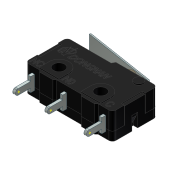
# Autodesk Inventor part: Microswitch Dongnan KW4A (S)
Saved by Autodesk Inventor 2015 (Build 190159000, 159)
## iProperties
Created: 2012-06-23
Part Number: Microswitch Dongnan KW4A (S)
Material: ABS Plastic
Document SubType Name: Modeling
Density: 1.06 g/cm^3
Mass: 1.24115 g
Surface Area: 16.0905 cm^2
Volume: 1.17089 cm^3
Appearance: Smooth - White
Categories: <MemberInstance><Categories><Category DisplayName="" Mnemonic="CABLEANDHARNESS" InternalName="e4a7e005-5e42-4d16-b293-125e7f0d0512"><Category DisplayName="" Mnemonic="CONNECTORS" InternalName="6f634eba-a678-4820-a31d-2c2d5ee6728e"><CategoryParameter DisplayName="" Mnemonic="REFDES" InternalName="c3740e8c-60ab-4d5d-8584-52b73222f2f0"/><Category DisplayName="" Mnemonic="DISCRETEWIRE" InternalName="9a3407de-09b2-4cdb-8c40-9708d5144a28"/></Category></Category></Categories><FamilyTemplate><FamilyTemplateParameters></FamilyTemplateParameters></FamilyTemplate><CategoryParameterMap><ParamToTemplateMap><ParamToTemplate CategoryParameter="//CategoryParameter[@InternalName='c3740e8c-60ab-4d5d-8584-52b73222f2f0']" ConstantValue=""/></ParamToTemplateMap></CategoryParameterMap></MemberInstance>
GlobalPropertyList: <PropertyList/>
Autodesk Inventor part; units mm, degrees
ref_plane "YZ Plane" through (0, 0, 0) normal (1, 0, 0) x (0, 1, 0)
ref_plane "XZ Plane" through (0, 0, 0) normal (0, 1, 0) x (-1, 0, 0)
ref_plane "XY Plane" through (0, 0, 0) normal (0, 0, 1) x (1, 0, 0)
sketch "Sketch1" plane through (0, 0, 0) normal (0, 0, 1) x (1, 0, 0)
  line L0 (-9.9, 5.1) -> (9.9, 5.1)
  line L1 (9.9, 5.1) -> (9.9, -5.1)
  line L2 (9.9, -5.1) -> (-9.9, -5.1)
  line L3 (-9.9, -5.1) -> (-9.9, 5.1)
  line L4 (-6.65, -5.1) -> (-6.25, -5.5)
  line L5 (-6.25, -5.5) -> (-3.25, -5.5)
  line L6 (-3.25, -5.5) -> (-2.85, -5.1)
  line L7 (2.85, -5.1) -> (3.25, -5.5)
  line L8 (3.25, -5.5) -> (6.25, -5.5)
  line L9 (6.25, -5.5) -> (6.65, -5.1)
  line L10 (-9.9, 4.4) -> (0.1, 4.4)
  line L11 (0.1, 4.4) -> (0.5041, 5.1)
  line L12 (4.75, -2.6) -> (-4.75, -2.6) construction
  circle A0 centre (-4.75, -2.6) radius 1.25
  circle A1 centre (4.75, -2.6) radius 1.25
  point P0 (0, 0)
  point P1 (0, 5.1)
  point P2 (9.9, 0)
  point P3 (0, -2.6)
  point P4 (-4.75, -5.5)
  point P5 (4.75, -5.5)
  dimension "d0" = 10.2
  dimension "d1" = 19.8
  dimension "d21" = 0.4
  dimension "d22" = 3
  dimension "d23" = 45
  dimension "d24" = 0.7
  dimension "d25" = 60
  dimension "d26" = 10
  dimension "d27" = 7.7
  dimension "d28" = 9.5
  dimension "d29" = 2.5
  constraints: 26 end point, 6 parallel, 6 point on line, 5 midpoint, 4 vertical alignment, 3 equal length, 2 centre point, 2 coincident, 2 horizontal alignment, 2 perpendicular, 1 collinear, 1 equal radius, 1 horizontal
  measures "d0" distance of L0.end L1.end
  measures "d1" distance of L0.start L0.end
  measures "d21" distance between parallel lines of L2 L8
  measures "d22" distance of L7.end L8.end
  measures "d23" angle of L8 L9
  measures "d24" distance between parallel lines of L0 L10
  measures "d25" angle of L10 L11
  measures "d26" distance of L10.start L10.end
  measures "d27" distance from line of L12.start L0
  measures "d28" distance of L12.start L12.end
  measures "d29" diameter of A0
extrude "Extrusion1" add sketch "Sketch1" along normal mid plane 6 contours L0 L1 L2 L3 L10 L11 | L2 L6 L5 L4 | L9 L8 L7 L2
sketch "Sketch3" plane through (0, 0, 3) normal (0, 0, 1) x (1, 0, 0)
  line L0 (-7, -4.85) -> (-7, -2.6)
  arc A0 (-2.5, -2.6) -> (-7, -2.6) centre (-4.75, -2.6) ccw
  line L1 (-2.5, -2.6) -> (-2.5, -4.85)
  line L2 (-7, -4.85) -> (-2.5, -4.85)
  circle A1 centre (-4.75, -2.6) radius 1.25 projected
  point P0 (0, 0)
  dimension "d13" = 4.5
  constraints: 6 end point, 3 tangent, 2 point on circle, 1 centre point, 1 coincident, 1 parallel, 1 perpendicular, 1 vertical
  measures "d13" distance of L0.start L1.end
extrude "Extrusion2" add sketch "Sketch3" along normal blind 0.25
sketch "Sketch17" plane through (0, 0, 3) normal (0, 0, 1) x (1, 0, 0)
  circle A0 centre (6.9, 3.9) radius 1
  line L0 (9.9, 5.1) -> (9.9, -5.1) projected
  line L1 (9.9, 5.1) -> (0.5041, 5.1) projected
  point P0 (0, 0)
  dimension "d126" = 2
  dimension "d128" = 3
  dimension "d129" = 1.2
  constraints: 1 centre point
  measures "d126" diameter of A0
  measures "d128" distance from line of L0 A0.centre
  measures "d129" distance from line of L1 A0.centre
extrude "Extrusion16" add sketch "Sketch17" along normal up to surface (0.25 mm away)
mirror "Mirror1" about plane through (0, 0, 0) normal (1, 0, 0) of "Extrusion2"
mirror "Mirror2" about plane through (0, 0, 0) normal (0, 0, 1) of "Extrusion2", "Mirror1", "Extrusion16"
sketch "Sketch5" plane through (-2.85, -5.1, 3) normal (0, -1, 0) x (1, 0, 0)
  line L0 (-5.55, -1.4) -> (-4.95, -1.4)
  line L1 (-4.95, -1.4) -> (-4.95, -4.6)
  line L2 (-4.95, -4.6) -> (-5.55, -4.6)
  line L3 (-5.55, -4.6) -> (-5.55, -1.4)
  line L4 (1.75, -1.4) -> (2.35, -1.4)
  line L5 (2.35, -1.4) -> (2.35, -4.6)
  line L6 (2.35, -4.6) -> (1.75, -4.6)
  line L7 (1.75, -4.6) -> (1.75, -1.4)
  line L8 (10.65, -1.4) -> (11.25, -1.4)
  line L9 (11.25, -1.4) -> (11.25, -4.6)
  line L10 (11.25, -4.6) -> (10.65, -4.6)
  line L11 (10.65, -4.6) -> (10.65, -1.4)
  line L12 (-7.05, -6) -> (-7.05, 0) projected
  line L13 (12.75, 0) -> (12.75, -6) projected
  point P0 (2.85, -3)
  point P1 (2.35, -3)
  point P2 (10.65, -3)
  point P3 (-4.95, -3)
  dimension "d30" = 0.6
  dimension "d31" = 3.2
  dimension "d32" = 1.5
  dimension "d33" = 8.8
  dimension "d34" = 1.5
  constraints: 24 end point, 6 parallel, 4 equal length, 3 horizontal, 3 horizontal alignment, 3 midpoint, 3 perpendicular
  measures "d30" distance of L0.start L0.end
  measures "d31" distance of L2.end L0.start
  measures "d32" distance between parallel lines of L12 L3
  measures "d33" distance between parallel lines of L12 L7
  measures "d34" distance between parallel lines of L13 L9
extrude "Extrusion4" add sketch "Sketch5" along normal blind 4.4 separate body
sketch "Sketch6" plane through (8.4, -5.1, 1.6) normal (1, 0, 0) x (0, 0, -1)
  line L0 (0, -4.4) -> (3.2, -4.4) projected
  line L1 (3.2, 0) -> (3.2, -4.4) projected
  line L2 (2.25, -4.4) -> (2.25, -0.9)
  line L3 (2.25, -0.9) -> (3.2, -0.9)
  point P0 (1.6, 5.1)
  dimension "d37" = 3.5
  dimension "d38" = 0.95
  constraints: 4 end point, 2 point on line, 1 parallel, 1 perpendicular
  measures "d37" distance between parallel lines of L0 L3
  measures "d38" distance between parallel lines of L1 L2
extrude "Extrusion5" cut sketch "Sketch6" against normal through all bodies 1 2
mirror "Mirror3" about plane through (0, 0, 0) normal (0, 0, 1) of "Extrusion5" bodies 2
full round fillet "Fillet1" bodies 2 first side at (8, -7.1667, -0.65) centre faces at (8, -9.5, 0.2167) second side at (8, -7.1667, 0.65)
full round fillet "Fillet2" bodies 2 first side at (-0.7, -8.3333, 0.65) centre faces at (-0.9, -9.5, 0.2167) second side at (-0.7, -8.3333, -0.65)
full round fillet "Fillet3" bodies 2 first side at (-8, -8.3333, -0.65) centre faces at (-8.2, -9.5, 0.2167) second side at (-8, -8.3333, 0.65)
fillet "Fillet4" radius 0.1 6 edges at (-8.1, -6, 0.65) (-0.8, -6, 0.65) (8.1, -6, 0.65) (8.1, -6, -0.65) (-0.8, -6, -0.65) (-8.1, -6, -0.65)
sketch "Sketch7" plane through (0, 0, 0) normal (0, 0, 1) x (1, 0, 0)
  line L0 (0.5041, 5.1) -> (9.9, 5.1) projected
  line L1 (1.9, 5.1) -> (1.9, 6.1)
  line L2 (3.9, 5.1) -> (3.9, 6.1)
  arc A0 (3.9, 6.1) -> (1.9, 6.1) centre (2.9, 5.5667) ccw
  line L3 (9.9, 5.1) -> (9.9, -5.1) projected
  point P0 (0, 0)
  dimension "d42" = 2
  dimension "d43" = 6
  dimension "d44" = 1.6
  dimension "d45" = 1
  constraints: 4 end point, 2 point on circle, 2 point on line, 1 centre point, 1 horizontal alignment, 1 parallel, 1 perpendicular
  measures "d42" distance between parallel lines of L1 L2
  measures "d43" distance between parallel lines of L3 L2
  measures "d45" distance of L2.start L2.end
extrude "Extrusion6" add sketch "Sketch7" along normal mid plane 3.6 separate body
sketch "Sketch8" plane through (0.5041, 5.1, 3) normal (0, 1, 0) x (1, 0, 0)
  line L0 (5.5959, 5.1) -> (6.5959, 5.1)
  line L1 (6.5959, 5.1) -> (6.5959, 0.9)
  line L2 (6.5959, 0.9) -> (5.5959, 0.9)
  line L3 (5.5959, 0.9) -> (5.5959, 5.1)
  line L4 (9.3959, 6) -> (9.3959, 0) projected
  point P0 (-0.5041, 3)
  point P1 (6.5959, 3)
  point P2 (9.3959, 3)
  dimension "d48" = 1
  dimension "d49" = 4.2
  dimension "d50" = 2.8
  constraints: 8 end point, 2 midpoint, 2 parallel, 1 horizontal, 1 horizontal alignment, 1 perpendicular
  measures "d48" distance of L0.start L0.end
  measures "d49" distance of L0.end L1.end
  measures "d50" distance between parallel lines of L4 L1
extrude "Extrusion7" cut sketch "Sketch8" against normal blind 1 bodies 1
sketch "Sketch9" plane through (0, 0, 0) normal (0, 0, 1) x (1, 0, 0)
  line L0 (6.9419, 4.1) -> (7.1997, 5.7305)
  line L1 (6.7008, 6.4169) -> (-9.0041, 8.9)
  line L2 (7.1, 4.1) -> (6.1, 4.1) projected
  arc A0 (7.1997, 5.7305) -> (6.7008, 6.4169) centre (6.6071, 5.8242) ccw
  line L3 (0.1, 4.4) -> (-9.9, 4.4) projected
  arc A1 (3.9, 6.1) -> (1.9, 6.1) centre (2.9, 5.5667) ccw projected
  point P0 (0, 0)
  point P1 (7.1, 5.1)
  dimension "d53" = 0.6
  dimension "d54" = 16.5
  dimension "d55" = 4.5
  dimension "d56" = 0.3
  constraints: 4 end point, 2 point on circle, 2 point on line, 2 tangent, 1 centre point, 1 perpendicular
  measures "d53" radius of A0
  measures "d54" distance from line of L1.end L0
  measures "d55" distance from line of L1.end L3
  measures "d56" distance edge to line of A1 L1
surface extrude "ExtrusionSrf1" sketch "Sketch9" along normal mid plane 4.1 shown no curves L0 A0 L1
thicken "Thicken1" operation new thickness 0.3 both sides no extend neighbours no toward (-0.9877298, 0.1561724, 0) faces at (7.0278, 4.6435, -0.6833) (7.1495, 6.0806, 0.6833) (1.4658, 7.2446, -0.6833)
fillet "Fillet5" radius 0.8 4 edges at (-9.9, 4.4, 0) (-9.9, -5.1, 0) (9.9, -5.1, 0) (9.9, 5.1, 0)
ref_plane "Work Plane1" through (0, 0, -1) normal (0, 0, 1) x (1, 0, 0)
split body "Split1" result two bodies by plane through (0, 0, -1) normal (0, 0, 1) bodies 1 first body at (-4.5331, 2.4803, -0.5)
sketch "Sketch10" plane through (0.1, 4.4, -1) normal (0, 0, -1) x (-1, 0, 0)
  line L0 (10, -8.7) -> (10, -0.8) projected
  line L1 (9.3, -2) -> (10, -2)
  line L2 (10, -2) -> (10, -6.8)
  line L3 (10, -6.8) -> (9.3, -6.8)
  line L4 (9.3, -6.8) -> (9.3, -2)
  line L5 (9.2, 0) -> (0, 0) projected
  point P0 (0.1, -4.4)
  dimension "d62" = 0.7
  dimension "d63" = 2
  dimension "d64" = 4.8
  constraints: 8 end point, 2 parallel, 1 horizontal, 1 perpendicular, 1 point on line
  measures "d62" distance between parallel lines of L2 L4
  measures "d63" distance between parallel lines of L5 L1
  measures "d64" distance of L3.end L1.start
extrude "Extrusion8" cut sketch "Sketch10" against normal through all bodies 5
sketch "Sketch11" plane through (0, 0, 0) normal (0, 1, 0) x (-1, 0, 0)
  line L0 (9.2, 0.1) -> (9.6, 0.1)
  line L1 (9.6, 0.1) -> (9.6, -0.7)
  line L2 (9.6, -0.7) -> (8.9, -2.2)
  line L3 (8.9, -2.2) -> (8.6, -2.2)
  line L4 (9.2, 3) -> (9.9, 3) projected
  line L5 (9.2, -1) -> (9.2, 3) projected
  line L6 (9.9, 3) -> (9.9, -1) projected
  line L7 (8.6, -2.2) -> (8.6, -1)
  line L8 (8.6, -1) -> (9.2, -1)
  point P0 (0, 0)
  dimension "d68" = 5.2
  dimension "d69" = 2.9
  dimension "d70" = 0.8
  dimension "d72" = 0.3
  dimension "d73" = 1
  dimension "d74" = 0.3
  constraints: 12 end point, 2 parallel, 1 perpendicular, 1 point on line, 1 vertical
  measures "d68" distance between parallel lines of L3 L4
  measures "d69" distance between parallel lines of L4 L0
  measures "d70" distance of L0.end L1.end
  measures "d72" distance between parallel lines of L1 L6
  measures "d73" distance from line of L6 L2.end
  measures "d74" distance of L2.end L3.end
extrude "Extrusion9" add sketch "Sketch11" along normal mid plane 1.3 bodies 5
sketch "Sketch12" plane through (-9.1, 4.4, -1) normal (0, 0, 1) x (1, 0, 0)
  line L0 (-0.8, -8.7) -> (-0.8, -0.8) projected
  line L1 (-0.8, -2.05) -> (-0.1, -2.05)
  line L2 (-0.1, -2.05) -> (-0.1, -6.75)
  line L3 (-0.1, -6.75) -> (-0.8, -6.75)
  line L4 (-0.8, -6.75) -> (-0.8, -2.05)
  line L5 (-0.5, -3.75) -> (-0.5, -5.05) projected
  point P0 (9.1, -4.4)
  point P1 (-0.1, -4.4)
  point P2 (-0.8, -4.4)
  point P3 (-0.5, -4.4)
  dimension "d77" = 0.7
  dimension "d78" = 4.7
  constraints: 8 end point, 3 midpoint, 2 horizontal alignment, 2 parallel, 1 horizontal, 1 perpendicular, 1 point on line
  measures "d77" distance of L1.start L1.end
  measures "d78" distance of L1.end L2.end
extrude "Extrusion10" add sketch "Sketch12" along normal blind 3.8 bodies 6
sketch "Sketch13" plane through (0, 0, -3) normal (0, 0, -1) x (-1, 0, 0)
  line L0 (9.9, 3.6) -> (9.9, -4.3) projected
  line L1 (9.9, 0.65) -> (8.9, 0.65)
  line L2 (8.9, 0.65) -> (8.9, -0.65)
  line L3 (8.9, -0.65) -> (9.9, -0.65)
  line L4 (9.9, -0.65) -> (9.9, 0.65)
  line L5 (9.9, -2.35) -> (9.9, 2.35) projected
  point P0 (0, 0)
  point P1 (9.9, 0)
  point P2 (9.9, -0.35)
  point P3 (9.9, 0)
  dimension "d81" = 1.3
  dimension "d82" = 1
  constraints: 8 end point, 3 midpoint, 2 parallel, 1 coincident, 1 horizontal, 1 perpendicular, 1 point on line
  measures "d81" distance of L1.end L2.end
  measures "d82" distance of L2.end L3.end
extrude "Extrusion11" cut sketch "Sketch13" against normal blind 3.1 bodies 6
sketch "Sketch14" plane through (-8.9, -0.65, -3) normal (-1, 0, 0) x (0, 0, 1)
  line L0 (2, 1.3) -> (2, 0) projected
  line L1 (0, 1.3) -> (2, 1.3) projected
  line L2 (0, 0) -> (0, 1.3) projected
  line L3 (0, 0) -> (2, 0) projected
  line L4 (2, 1.3) -> (0.7, 1.3)
  line L5 (0.7, 1.3) -> (0.7, 0)
  line L6 (0.7, 0) -> (2, 0)
  line L7 (2, 0) -> (2, 1.3)
  point P0 (3, 0.65)
  dimension "d85" = 0.7
  constraints: 8 end point, 2 parallel, 1 horizontal, 1 perpendicular, 1 point on line
  measures "d85" distance between parallel lines of L2 L5
extrude "Extrusion12" cut sketch "Sketch14" against normal blind 1 contours L0 L3 L5 L1 bodies 6
mirror "Mirror4" about plane through (0, 0, 0) normal (1, 0, 0) of "Extrusion8", "Extrusion9" bodies 5
mirror "Mirror5" about plane through (0, 0, 0) normal (1, 0, 0) of "Extrusion10", "Extrusion11", "Extrusion12" bodies 6
sketch "Sketch15" plane through (0, 0, 3) normal (0, 0, 1) x (1, 0, 0)
  line L0 (-9.6, -3.1) -> (-7.0718, -3.1) construction
  line L1 (-7.0718, -3.1) -> (-7.0718, -5.3594) construction
  line L2 (-7.0718, -5.3594) -> (-9.6, -5.3594) construction
  line L3 (-9.6, -5.3594) -> (-9.6, -3.1) construction
  line L4 (-2.3, -3.1) -> (0.2282, -3.1) construction
  line L5 (0.2282, -3.1) -> (0.2282, -5.3594) construction
  line L6 (0.2282, -5.3594) -> (-2.3, -5.3594) construction
  line L7 (-2.3, -5.3594) -> (-2.3, -3.1) construction
  line L8 (7.5, -5.3594) -> (7.5, -3.1) construction
  line L9 (7.5, -3.1) -> (10.0282, -3.1) construction
  line L10 (10.0282, -3.1) -> (10.0282, -5.3594) construction
  line L11 (10.0282, -5.3594) -> (7.5, -5.3594) construction
  line L12 (-6.65, -5.1) -> (-9.1, -5.1) projected
  line L13 (-9.9, -4.3) -> (-9.9, -2.4) projected
  line L14 (-6.1061, 1.9) -> (2.8193, 1.9) construction
  line L15 (2.8193, 1.9) -> (2.8193, 0.5) construction
  line L16 (2.8193, 0.5) -> (-6.1061, 0.5) construction
  line L17 (-6.1061, 0.5) -> (-6.1061, 1.9) construction
  line L18 (-8.2, 0.6) -> (-7.85, 0.6)
  line L19 (-7.85, 0.6) -> (-7.5869, 2.0924)
  line L20 (-7.5869, 2.0924) -> (-7.3061, 0.5)
  line L21 (-7.3061, 0.5) -> (-6.8061, 0.5)
  line L22 (-6.8061, 0.5) -> (-6.5436, 3.5)
  line L23 (-6.5436, 3.5) -> (-7.0746, 1.2)
  line L24 (-7.0746, 1.2) -> (-7.5569, 3)
  line L25 (-7.5569, 3) -> (-8.2, 0.6)
  arc A0 (-6.5495, 2.7981) -> (-8.3, 1.85) centre (-6.3326, 0.3075) ccw
  arc A1 (-6.0803, 2.0379) -> (-6.5495, 2.7981) centre (-6.5061, 2.3) ccw
  arc A2 (-8.3, 0.85) -> (-6.0803, 2.0379) centre (-8.2093, 3.3484) ccw
  line L26 (-8.3, 1.85) -> (-8.3, 0.85)
  arc A3 (-6.5581, 2.8977) -> (-8.4, 1.8841) centre (-6.3326, 0.3075) ccw
  arc A4 (-5.9951, 1.9855) -> (-6.5581, 2.8977) centre (-6.5061, 2.3) ccw
  arc A5 (-8.4, 0.7554) -> (-5.9951, 1.9855) centre (-8.2093, 3.3484) ccw
  line L27 (-8.4, 0.7554) -> (-8.4, 1.8841)
  line L28 (-9.2, 2.4) -> (-9.2, -2.4) projected
  line L29 (-9.472, -4.6263) -> (-9.472, -3.1263)
  line L30 (-9.472, -3.1263) -> (-9.3096, -3.1263)
  line L31 (-9.3096, -3.1263) -> (-8.6785, -4.3039)
  line L32 (-8.6785, -4.3039) -> (-8.6785, -3.1263)
  line L33 (-8.6785, -3.1263) -> (-8.5264, -3.1263)
  line L34 (-8.5264, -3.1263) -> (-8.5264, -4.6263)
  line L35 (-8.5264, -4.6263) -> (-8.6888, -4.6263)
  line L36 (-8.6888, -4.6263) -> (-9.3199, -3.4487)
  line L37 (-9.3199, -3.4487) -> (-9.3199, -4.6263)
  line L38 (-9.3199, -4.6263) -> (-9.472, -4.6263)
  line L39 (-7.4049, -4.0992) -> (-7.246, -4.1495)
  spline S0 degree 2 poles (-7.246, -4.1495) (-7.2963, -4.3942) (-7.5558, -4.6514) (-7.7433, -4.6514) knots 0 0 0 1 2 2 2
  spline S1 degree 2 poles (-7.7433, -4.6514) (-7.9365, -4.6514) (-8.18, -4.4537) (-8.3069, -4.0798) (-8.3069, -3.8649) knots 0 0 0 1 2 3 3 3
  spline S2 degree 2 poles (-8.3069, -3.8649) (-8.3069, -3.6305) (-8.164, -3.2806) (-7.8988, -3.1) (-7.741, -3.1) knots 0 0 0 1 2 3 3 3
  spline S3 degree 2 poles (-7.741, -3.1) (-7.5604, -3.1) (-7.3146, -3.3298) (-7.2665, -3.5367) knots 0 0 0 1 2 2 2
  line L40 (-7.2665, -3.5367) -> (-7.4232, -3.5836)
  spline S4 degree 2 poles (-7.4232, -3.5836) (-7.4655, -3.4201) (-7.6232, -3.2704) (-7.7444, -3.2704) knots 0 0 0 1 2 2 2
  spline S5 degree 2 poles (-7.7444, -3.2704) (-7.8828, -3.2704) (-8.068, -3.4361) (-8.1434, -3.7151) (-8.1434, -3.8637) knots 0 0 0 1 2 3 3 3
  spline S6 degree 2 poles (-8.1434, -3.8637) (-8.1434, -4.0546) (-8.0543, -4.3405) (-7.8656, -4.4811) (-7.7559, -4.4811) knots 0 0 0 1 2 3 3 3
  spline S7 degree 2 poles (-7.7559, -4.4811) (-7.6221, -4.4811) (-7.438, -4.289) (-7.4049, -4.0992) knots 0 0 0 1 2 2 2
  line L41 (-2.172, -4.6057) -> (-2.172, -3.1057)
  line L42 (-2.172, -3.1057) -> (-2.0096, -3.1057)
  line L43 (-2.0096, -3.1057) -> (-1.3785, -4.2833)
  line L44 (-1.3785, -4.2833) -> (-1.3785, -3.1057)
  line L45 (-1.3785, -3.1057) -> (-1.2264, -3.1057)
  line L46 (-1.2264, -3.1057) -> (-1.2264, -4.6057)
  line L47 (-1.2264, -4.6057) -> (-1.3888, -4.6057)
  line L48 (-1.3888, -4.6057) -> (-2.0199, -3.4281)
  line L49 (-2.0199, -3.4281) -> (-2.0199, -4.6057)
  line L50 (-2.0199, -4.6057) -> (-2.172, -4.6057)
  spline S8 degree 2 poles (-1.0207, -3.866) (-1.0207, -3.5996) (-0.9326, -3.2749) (-0.76, -3.1) (-0.6296, -3.1) knots 0 0 0 1 2 3 3 3
  spline S9 degree 2 poles (-0.6296, -3.1) (-0.5336, -3.1) (-0.3873, -3.1972) (-0.2924, -3.3801) (-0.2386, -3.6431) (-0.2386, -3.866) knots 0 0 0 1 2 3 4 4 4
  spline S10 degree 2 poles (-0.2386, -3.866) (-0.2386, -4.1301) (-0.3255, -4.4548) (-0.4982, -4.6309) (-0.6296, -4.6309) knots 0 0 0 1 2 3 3 3
  spline S11 degree 2 poles (-0.6296, -4.6309) (-0.8034, -4.6309) (-0.9018, -4.4765) knots 0 0 0 1 1 1
  spline S12 degree 2 poles (-0.9018, -4.4765) (-1.0207, -4.2879) (-1.0207, -3.866) knots 0 0 0 1 1 1
  spline S13 degree 2 poles (-0.8697, -3.866) (-0.8697, -4.2364) (-0.7314, -4.48) (-0.6296, -4.48) knots 0 0 0 1 2 2 2
  spline S14 degree 2 poles (-0.6296, -4.48) (-0.5279, -4.48) (-0.3896, -4.2353) (-0.3896, -3.866) knots 0 0 0 1 2 2 2
  spline S15 degree 2 poles (-0.3896, -3.866) (-0.3896, -3.4956) (-0.5279, -3.2521) (-0.6308, -3.2521) knots 0 0 0 1 2 2 2
  spline S16 degree 2 poles (-0.6308, -3.2521) (-0.7325, -3.2521) (-0.7943, -3.3595) knots 0 0 0 1 1 1
  spline S17 degree 2 poles (-0.7943, -3.3595) (-0.8697, -3.4967) (-0.8697, -3.866) knots 0 0 0 1 1 1
  spline S18 degree 2 poles (-4.6762, 1.1955) (-4.7386, 1.0106) (-4.9891, 0.713) (-5.1434, 0.6299) knots 0 0 0 1 2 2 2
  spline S19 degree 2 poles (-5.1434, 0.6299) (-5.2681, 0.5653) (-5.4945, 0.5216) (-5.6586, 0.5216) knots 0 0 0 1 2 2 2
  line L51 (-5.6586, 0.5216) -> (-5.9693, 0.5216)
  line L52 (-5.9693, 0.5216) -> (-5.5109, 1.8716)
  line L53 (-5.5109, 1.8716) -> (-5.2035, 1.8716)
  spline S20 degree 2 poles (-5.2035, 1.8716) (-5.0132, 1.8716) (-4.8152, 1.8147) (-4.7561, 1.7643) knots 0 0 0 1 2 2 2
  spline S21 degree 2 poles (-4.7561, 1.7643) (-4.6554, 1.6779) (-4.6084, 1.3924) (-4.6762, 1.1955) knots 0 0 0 1 2 2 2
  spline S22 degree 2 poles (-4.8622, 1.1976) (-4.8097, 1.353) (-4.8381, 1.5729) (-4.918, 1.6353) knots 0 0 0 1 2 2 2
  spline S23 degree 2 poles (-4.918, 1.6353) (-4.9749, 1.6779) (-5.1259, 1.7162) (-5.2473, 1.7162) knots 0 0 0 1 2 2 2
  line L54 (-5.2473, 1.7162) -> (-5.384, 1.7162)
  line L55 (-5.384, 1.7162) -> (-5.7374, 0.6769)
  line L56 (-5.7374, 0.6769) -> (-5.6007, 0.6769)
  spline S24 degree 2 poles (-5.6007, 0.6769) (-5.4803, 0.6769) (-5.2878, 0.7152) (-5.1959, 0.7666) knots 0 0 0 1 2 2 2
  spline S25 degree 2 poles (-5.1959, 0.7666) (-5.081, 0.8301) (-4.9158, 1.0401) (-4.8622, 1.1976) knots 0 0 0 1 2 2 2
  spline S26 degree 2 poles (-3.3492, 1.7173) (-3.3022, 1.6276) (-3.3065, 1.365) (-3.3634, 1.1966) knots 0 0 0 1 2 2 2
  spline S27 degree 2 poles (-3.3634, 1.1966) (-3.4192, 1.0325) (-3.5932, 0.7666) (-3.7026, 0.6769) knots 0 0 0 1 2 2 2
  spline S28 degree 2 poles (-3.7026, 0.6769) (-3.8174, 0.5828) (-4.068, 0.4931) (-4.2003, 0.4931) knots 0 0 0 1 2 2 2
  spline S29 degree 2 poles (-4.2003, 0.4931) (-4.3371, 0.4931) (-4.5252, 0.5861) (-4.5723, 0.6769) knots 0 0 0 1 2 2 2
  spline S30 degree 2 poles (-4.5723, 0.6769) (-4.6204, 0.7666) (-4.6139, 1.0303) (-4.557, 1.1966) knots 0 0 0 1 2 2 2
  spline S31 degree 2 poles (-4.557, 1.1966) (-4.499, 1.3661) (-4.3272, 1.6243) (-4.2178, 1.7173) knots 0 0 0 1 2 2 2
  spline S32 degree 2 poles (-4.2178, 1.7173) (-4.1095, 1.807) (-3.8579, 1.9) (-3.7222, 1.9) knots 0 0 0 1 2 2 2
  spline S33 degree 2 poles (-3.7222, 1.9) (-3.5844, 1.9) (-3.3962, 1.8037) (-3.3492, 1.7173) knots 0 0 0 1 2 2 2
  spline S34 degree 2 poles (-3.5505, 1.1966) (-3.5056, 1.33) (-3.4936, 1.5368) (-3.522, 1.6046) knots 0 0 0 1 2 2 2
  spline S35 degree 2 poles (-3.522, 1.6046) (-3.5527, 1.6746) (-3.6796, 1.7447) (-3.7737, 1.7447) knots 0 0 0 1 2 2 2
  spline S36 degree 2 poles (-3.7737, 1.7447) (-3.8721, 1.7447) (-4.0406, 1.6768) (-4.1205, 1.6046) knots 0 0 0 1 2 2 2
  spline S37 degree 2 poles (-4.1205, 1.6046) (-4.1981, 1.5357) (-4.3261, 1.3278) (-4.3699, 1.1966) knots 0 0 0 1 2 2 2
  spline S38 degree 2 poles (-4.3699, 1.1966) (-4.4607, 0.9307) (-4.3338, 0.6485) (-4.1467, 0.6485) knots 0 0 0 1 2 2 2
  spline S39 degree 2 poles (-4.1467, 0.6485) (-3.9586, 0.6485) (-3.6413, 0.9307) (-3.5505, 1.1966) knots 0 0 0 1 2 2 2
  line L57 (-2.4302, 0.5216) -> (-2.6315, 0.5216)
  line L58 (-2.6315, 0.5216) -> (-2.8328, 1.6856)
  line L59 (-2.8328, 1.6856) -> (-3.2289, 0.5216)
  line L60 (-3.2289, 0.5216) -> (-3.3962, 0.5216)
  line L61 (-3.3962, 0.5216) -> (-2.9378, 1.8716)
  line L62 (-2.9378, 1.8716) -> (-2.6829, 1.8716)
  line L63 (-2.6829, 1.8716) -> (-2.5024, 0.8027)
  line L64 (-2.5024, 0.8027) -> (-2.1392, 1.8716)
  line L65 (-2.1392, 1.8716) -> (-1.9718, 1.8716)
  line L66 (-1.9718, 1.8716) -> (-2.4302, 0.5216)
  spline S40 degree 2 poles (-1.5999, 0.4953) (-1.7432, 0.4953) (-1.9511, 0.5828) (-2.0069, 0.6714) knots 0 0 0 1 2 2 2
  spline S41 degree 2 poles (-2.0069, 0.6714) (-2.0616, 0.7611) (-2.0616, 1.0259) (-2.0036, 1.1976) knots 0 0 0 1 2 2 2
  spline S42 degree 2 poles (-2.0036, 1.1976) (-1.9478, 1.3607) (-1.7684, 1.6188) (-1.6524, 1.7107) knots 0 0 0 1 2 2 2
  spline S43 degree 2 poles (-1.6524, 1.7107) (-1.5397, 1.7994) (-1.2662, 1.8956) (-1.1229, 1.8956) knots 0 0 0 1 2 2 2
  spline S44 degree 2 poles (-1.1229, 1.8956) (-1.0551, 1.8956) (-0.9358, 1.8759) (-0.8855, 1.8584) knots 0 0 0 1 2 2 2
  spline S45 degree 2 poles (-0.8855, 1.8584) (-0.8439, 1.8453) (-0.7487, 1.7972) (-0.7203, 1.7797) knots 0 0 0 1 2 2 2
  line L67 (-0.7203, 1.7797) -> (-0.7936, 1.563)
  line L68 (-0.7936, 1.563) -> (-0.81, 1.563)
  spline S46 degree 2 poles (-0.81, 1.563) (-0.833, 1.5926) (-0.8866, 1.6462) (-0.9413, 1.6768) knots 0 0 0 1 2 2 2
  spline S47 degree 2 poles (-0.9413, 1.6768) (-0.9861, 1.7042) (-1.1152, 1.7403) (-1.1973, 1.7403) knots 0 0 0 1 2 2 2
  spline S48 degree 2 poles (-1.1973, 1.7403) (-1.392, 1.7403) (-1.7323, 1.4471) (-1.8143, 1.2031) knots 0 0 0 1 2 2 2
  spline S49 degree 2 poles (-1.8143, 1.2031) (-1.8603, 1.0675) (-1.8657, 0.864) (-1.8307, 0.794) knots 0 0 0 1 2 2 2
  spline S50 degree 2 poles (-1.8307, 0.794) (-1.7957, 0.7239) (-1.6568, 0.6506) (-1.5539, 0.6506) knots 0 0 0 1 2 2 2
  spline S51 degree 2 poles (-1.5539, 0.6506) (-1.4784, 0.6506) (-1.3198, 0.6725) (-1.2607, 0.6944) knots 0 0 0 1 2 2 2
  line L69 (-1.2607, 0.6944) -> (-1.1426, 1.0434)
  line L70 (-1.1426, 1.0434) -> (-1.4555, 1.0434)
  line L71 (-1.4555, 1.0434) -> (-1.4019, 1.2009)
  line L72 (-1.4019, 1.2009) -> (-0.9118, 1.2009)
  line L73 (-0.9118, 1.2009) -> (-1.112, 0.6113)
  spline S52 degree 2 poles (-1.112, 0.6113) (-1.1513, 0.5959) (-1.2826, 0.5489) (-1.3373, 0.5347) knots 0 0 0 1 2 2 2
  spline S53 degree 2 poles (-1.3373, 0.5347) (-1.4106, 0.515) (-1.5244, 0.4953) (-1.5999, 0.4953) knots 0 0 0 1 2 2 2
  line L74 (0.0488, 0.5216) -> (-0.1525, 0.5216)
  line L75 (-0.1525, 0.5216) -> (-0.3538, 1.6856)
  line L76 (-0.3538, 1.6856) -> (-0.7498, 0.5216)
  line L77 (-0.7498, 0.5216) -> (-0.9172, 0.5216)
  line L78 (-0.9172, 0.5216) -> (-0.4588, 1.8716)
  line L79 (-0.4588, 1.8716) -> (-0.2039, 1.8716)
  line L80 (-0.2039, 1.8716) -> (-0.0234, 0.8027)
  line L81 (-0.0234, 0.8027) -> (0.3398, 1.8716)
  line L82 (0.3398, 1.8716) -> (0.5072, 1.8716)
  line L83 (0.5072, 1.8716) -> (0.0488, 0.5216)
  line L84 (0.1768, 0.5216) -> (1.0903, 1.8716)
  line L85 (1.0903, 1.8716) -> (1.3113, 1.8716)
  line L86 (1.3113, 1.8716) -> (1.308, 0.5216)
  line L87 (1.308, 0.5216) -> (1.1187, 0.5216)
  line L88 (1.1187, 0.5216) -> (1.1242, 0.899)
  line L89 (1.1242, 0.899) -> (0.6089, 0.899)
  line L90 (0.6089, 0.899) -> (0.3584, 0.5216)
  line L91 (0.3584, 0.5216) -> (0.1768, 0.5216)
  line L92 (1.1264, 1.0521) -> (1.134, 1.6878)
  line L93 (1.134, 1.6878) -> (0.7107, 1.0521)
  line L94 (0.7107, 1.0521) -> (1.1264, 1.0521)
  line L95 (2.402, 0.5216) -> (2.2007, 0.5216)
  line L96 (2.2007, 0.5216) -> (1.9994, 1.6856)
  line L97 (1.9994, 1.6856) -> (1.6034, 0.5216)
  line L98 (1.6034, 0.5216) -> (1.436, 0.5216)
  line L99 (1.436, 0.5216) -> (1.8944, 1.8716)
  line L100 (1.8944, 1.8716) -> (2.1493, 1.8716)
  line L101 (2.1493, 1.8716) -> (2.3298, 0.8027)
  line L102 (2.3298, 0.8027) -> (2.693, 1.8716)
  line L103 (2.693, 1.8716) -> (2.8604, 1.8716)
  line L104 (2.8604, 1.8716) -> (2.402, 0.5216)
  line L105 (8.4855, -4.0992) -> (8.6444, -4.1495)
  spline S54 degree 2 poles (8.6444, -4.1495) (8.5941, -4.3942) (8.3346, -4.6514) (8.1471, -4.6514) knots 0 0 0 1 2 2 2
  spline S55 degree 2 poles (8.1471, -4.6514) (7.9539, -4.6514) (7.7104, -4.4537) (7.5835, -4.0798) (7.5835, -3.8649) knots 0 0 0 1 2 3 3 3
  spline S56 degree 2 poles (7.5835, -3.8649) (7.5835, -3.6305) (7.7264, -3.2806) (7.9916, -3.1) (8.1494, -3.1) knots 0 0 0 1 2 3 3 3
  spline S57 degree 2 poles (8.1494, -3.1) (8.33, -3.1) (8.5758, -3.3298) (8.6239, -3.5367) knots 0 0 0 1 2 2 2
  line L106 (8.6239, -3.5367) -> (8.4672, -3.5836)
  spline S58 degree 2 poles (8.4672, -3.5836) (8.4249, -3.4201) (8.2671, -3.2704) (8.146, -3.2704) knots 0 0 0 1 2 2 2
  spline S59 degree 2 poles (8.146, -3.2704) (8.0076, -3.2704) (7.8224, -3.4361) (7.747, -3.7151) (7.747, -3.8637) knots 0 0 0 1 2 3 3 3
  spline S60 degree 2 poles (7.747, -3.8637) (7.747, -4.0546) (7.8361, -4.3405) (8.0248, -4.4811) (8.1345, -4.4811) knots 0 0 0 1 2 3 3 3
  spline S61 degree 2 poles (8.1345, -4.4811) (8.2683, -4.4811) (8.4524, -4.289) (8.4855, -4.0992) knots 0 0 0 1 2 2 2
  point P0 (0, 0)
  dimension "d88" = 2
  dimension "d89" = 0.3
  dimension "d90" = 7.6
  dimension "d91" = 17.4
  dimension "d92" = 0.5
  dimension "d93" = 0.35
  dimension "d94" = 0.1
  dimension "d95" = 95
  dimension "d96" = 3
  dimension "d97" = 8
  dimension "d99" = 100
  dimension "d100" = 100
  dimension "d101" = 75
  dimension "d102" = 0.7
  dimension "d103" = 0.5
  dimension "d104" = 28
  dimension "d105" = 1.4
  dimension "d106" = 0.7
  dimension "d107" = 1.8
  dimension "d108" = 0.5
  dimension "d109" = 2.5
  dimension "d110" = 2.5
  dimension "d111" = 0.1
  dimension "d112" = 1
  dimension "d113" = 0.35
  dimension "d114" = 0.3
  dimension "d115" = 0.1
  dimension "d116" = 0.8
  dimension "d117" = 5.6
  constraints: 20 end point, 12 point on circle, 6 centre point, 3 horizontal alignment, 2 perpendicular, 2 tangent, 1 horizontal, 1 parallel, 11 other
  measures "d88" distance between parallel lines of L12 L0
  measures "d89" distance between parallel lines of L3 L13
  measures "d90" distance between parallel lines of L13 L7
  measures "d91" distance between parallel lines of L13 L8
  measures "d92" distance of L20.end L21.end
  measures "d93" distance of L18.start L18.end
  measures "d94" distance between parallel lines of L18 L21
  measures "d95" angle of L22 L21
  measures "d96" distance from line of L22.end L21
  measures "d97" angle of L22 L23
  measures "d99" angle of L21 L20
  measures "d100" angle of L18 L19
  measures "d101" angle of L18 L25
  measures "d102" distance from line of L21 L23.end
  measures "d103" vertical distance of L24.end L22.end
  measures "d104" angle of L23 L24
  measures "d105" distance of L16.end L14.start
  measures "d106" distance from line of L21.end L17
  measures "d107" distance from line of L21 A1.centre
  measures "d108" radius of A1
  measures "d109" radius of A0
  measures "d110" radius of A2
  measures "d111" distance from line of L18.start L26
  measures "d112" distance of L26.start L26.end
  measures "d113" distance from line of L21 L26.end
  measures "d114" horizontal distance of L21.end A1.centre
  measures "d115" radial gap between concentric circles of A1 A4
  measures "d116" distance between parallel lines of L28 L27
  measures "d117" distance between parallel lines of L12 L16
extrude "Extrusion13" add sketch "Sketch15" along normal blind 0.1 contours L25 A5 L19 L18 | A5 L27 A3 L25 A0 L26 A2 | L25 A2 L19 A5 | L19 A2 L20 A5 | L25 A0 L24 L23 L22 A2 L20 L19 | A5 L22 L21 L20 | L20 A2 L22 A5 | L25 A3 L24 A0 | L22 A2 A1 A0 A3 A4 A5 | L25 L24 A3 | L24 A3 L23 A0 | L23 A3 L22 A0 | L23 L22 A3 | L29 L30 L31 L32 L33 L34 L35 L36 L37 L38 | L39 S0 S1 S2 S3 L40 S4 S5 S6 S7 | L41 L42 L43 L44 L45 L46 L47 L48 L49 L50 | S8 S9 S10 S11 S12 | S18 S19 L51 L52 L53 S20 S21 | S26 S27 S28 S29 S30 S31 S32 S33 | L57 L58 L59 L60 L61 L62 L63 L64 L65 L66 | S40 S41 S42 S43 S44 S45 L67 L68 S46 S47 S48 S49 S50 S51 L69 L70 L71 L72 L73 S52 S53 | L74 L75 L76 L77 L78 L79 L80 L81 L82 L83 | L84 L85 L86 L87 L88 L89 L90 L91 | L95 L96 L97 L98 L99 L100 L101 L102 L103 L104 | L105 S54 S55 S56 S57 L106 S58 S59 S60 S61 bodies 5
extrude "Extrusion14" add sketch "Sketch15" along normal up to surface (0.1 mm away) contours L25 A5 L19 L18 | L25 A2 L19 A5 | L25 A0 L24 L23 L22 A2 L20 L19 | A5 L22 L21 L20 | L20 A2 L22 A5 | L25 A3 L24 A0 | L25 L24 A3 | L23 A3 L22 A0 | L23 L22 A3 bodies 5
sketch "Sketch16" plane through (0, 0, -3) normal (0, 0, -1) x (-1, 0, 0)
  line L0 (-5.4, 4.6) -> (15.1547, 4.6) construction
  line L1 (15.1547, 4.6) -> (15.1547, -0.0232) construction
  line L2 (15.1547, -0.0232) -> (-5.4, -0.0232) construction
  line L3 (-5.4, -0.0232) -> (-5.4, 4.6) construction
  line L4 (-9.1, 5.1) -> (-0.5041, 5.1) projected
  line L5 (-9.9, 0.65) -> (-9.9, 4.3) projected
  line L6 (-4.7363, 3.5554) -> (-4.8741, 3.5554)
  line L7 (-4.8741, 3.5554) -> (-5.1658, 4.0206)
  line L8 (-5.1658, 4.0206) -> (-5.2128, 3.9549)
  line L9 (-5.2128, 3.9549) -> (-5.2128, 3.5554)
  line L10 (-5.2128, 3.5554) -> (-5.319, 3.5554)
  line L11 (-5.319, 3.5554) -> (-5.319, 4.5554)
  line L12 (-5.319, 4.5554) -> (-5.2128, 4.5554)
  line L13 (-5.2128, 4.5554) -> (-5.2128, 4.0951)
  line L14 (-5.2128, 4.0951) -> (-4.8854, 4.5554)
  line L15 (-4.8854, 4.5554) -> (-4.7558, 4.5554)
  line L16 (-4.7558, 4.5554) -> (-5.0864, 4.1089)
  line L17 (-5.0864, 4.1089) -> (-4.7363, 3.5554)
  line L18 (-3.7752, 4.5554) -> (-3.9762, 3.5554)
  line L19 (-3.9762, 3.5554) -> (-4.0961, 3.5554)
  line L20 (-4.0961, 3.5554) -> (-4.259, 4.3853)
  line L21 (-4.259, 4.3853) -> (-4.4178, 3.5554)
  line L22 (-4.4178, 3.5554) -> (-4.5345, 3.5554)
  line L23 (-4.5345, 3.5554) -> (-4.7395, 4.5554)
  line L24 (-4.7395, 4.5554) -> (-4.6301, 4.5554)
  line L25 (-4.6301, 4.5554) -> (-4.4689, 3.724)
  line L26 (-4.4689, 3.724) -> (-4.3092, 4.5554)
  line L27 (-4.3092, 4.5554) -> (-4.2015, 4.5554)
  line L28 (-4.2015, 4.5554) -> (-4.0394, 3.7159)
  line L29 (-4.0394, 3.7159) -> (-3.8797, 4.5554)
  line L30 (-3.8797, 4.5554) -> (-3.7752, 4.5554)
  line L31 (-3.1885, 3.899) -> (-3.2833, 3.899)
  line L32 (-3.2833, 3.899) -> (-3.2833, 3.5554)
  line L33 (-3.2833, 3.5554) -> (-3.3862, 3.5554)
  line L34 (-3.3862, 3.5554) -> (-3.3862, 3.899)
  line L35 (-3.3862, 3.899) -> (-3.7395, 3.899)
  line L36 (-3.7395, 3.899) -> (-3.7395, 4.04)
  line L37 (-3.7395, 4.04) -> (-3.3822, 4.5554)
  line L38 (-3.3822, 4.5554) -> (-3.2833, 4.5554)
  line L39 (-3.2833, 4.5554) -> (-3.2833, 4.0068)
  line L40 (-3.2833, 4.0068) -> (-3.1885, 4.0068)
  line L41 (-3.1885, 4.0068) -> (-3.1885, 3.899)
  line L42 (-3.3862, 4.0068) -> (-3.3862, 4.3966)
  line L43 (-3.3862, 4.3966) -> (-3.6561, 4.0068)
  line L44 (-3.6561, 4.0068) -> (-3.3862, 4.0068)
  line L45 (-3.1666, 3.5554) -> (-2.8968, 4.5554)
  line L46 (-2.8968, 4.5554) -> (-2.7655, 4.5554)
  line L47 (-2.7655, 4.5554) -> (-2.4956, 3.5554)
  line L48 (-2.4956, 3.5554) -> (-2.6075, 3.5554)
  line L49 (-2.6075, 3.5554) -> (-2.6796, 3.835)
  line L50 (-2.6796, 3.835) -> (-2.9867, 3.835)
  line L51 (-2.9867, 3.835) -> (-3.0588, 3.5554)
  line L52 (-3.0588, 3.5554) -> (-3.1666, 3.5554)
  line L53 (-2.7096, 3.9485) -> (-2.8335, 4.4217)
  line L54 (-2.8335, 4.4217) -> (-2.9567, 3.9485)
  line L55 (-2.9567, 3.9485) -> (-2.7096, 3.9485)
  line L56 (-1.776, 3.2791) -> (-1.8992, 3.2791)
  spline S0 degree 2 poles (-1.8992, 3.2791) (-1.9924, 3.4177) (-2.0994, 3.728) (-2.0994, 3.9395) knots 0 0 0 1 2 2 2
  spline S1 degree 2 poles (-2.0994, 3.9395) (-2.0994, 4.1462) (-1.9932, 4.4614) (-1.8992, 4.6) knots 0 0 0 1 2 2 2
  line L57 (-1.8992, 4.6) -> (-1.776, 4.6)
  line L58 (-1.776, 4.6) -> (-1.776, 4.5935)
  spline S2 degree 2 poles (-1.776, 4.5935) (-1.8198, 4.5441) (-1.8984, 4.416) (-1.9324, 4.331) knots 0 0 0 1 2 2 2
  spline S3 degree 2 poles (-1.9324, 4.331) (-1.964, 4.2483) (-2.0045, 4.0498) (-2.0045, 3.9395) knots 0 0 0 1 2 2 2
  spline S4 degree 2 poles (-2.0045, 3.9395) (-2.0045, 3.8245) (-1.9656, 3.634) (-1.9324, 3.5481) knots 0 0 0 1 2 2 2
  spline S5 degree 2 poles (-1.9324, 3.5481) (-1.9, 3.4655) (-1.8173, 3.3318) (-1.776, 3.2856) knots 0 0 0 1 2 2 2
  line L59 (-1.776, 3.2856) -> (-1.776, 3.2791)
  spline S6 degree 2 poles (-1.4324, 3.5376) (-1.5191, 3.5376) (-1.6415, 3.583) (-1.695, 3.6154) knots 0 0 0 1 2 2 2
  line L60 (-1.695, 3.6154) -> (-1.695, 3.7823)
  line L61 (-1.695, 3.7823) -> (-1.6877, 3.7823)
  spline S7 degree 2 poles (-1.6877, 3.7823) (-1.635, 3.7207) (-1.5013, 3.6527) (-1.4397, 3.6527) knots 0 0 0 1 2 2 2
  spline S8 degree 2 poles (-1.4397, 3.6527) (-1.3514, 3.6527) (-1.2614, 3.7442) (-1.2614, 3.8196) knots 0 0 0 1 2 2 2
  spline S9 degree 2 poles (-1.2614, 3.8196) (-1.2614, 3.8796) (-1.3092, 3.9541) (-1.3603, 3.9728) knots 0 0 0 1 2 2 2
  spline S10 degree 2 poles (-1.3603, 3.9728) (-1.3976, 3.9857) (-1.4592, 4.0036) (-1.5053, 4.0182) knots 0 0 0 1 2 2 2
  spline S11 degree 2 poles (-1.5053, 4.0182) (-1.5467, 4.0319) (-1.6123, 4.0733) (-1.6374, 4.1065) knots 0 0 0 1 2 2 2
  spline S12 degree 2 poles (-1.6374, 4.1065) (-1.6618, 4.1397) (-1.6893, 4.2288) (-1.6893, 4.2872) knots 0 0 0 1 2 2 2
  spline S13 degree 2 poles (-1.6893, 4.2872) (-1.6893, 4.4088) (-1.5378, 4.5733) (-1.4203, 4.5733) knots 0 0 0 1 2 2 2
  spline S14 degree 2 poles (-1.4203, 4.5733) (-1.353, 4.5733) (-1.2331, 4.54) (-1.182, 4.5084) knots 0 0 0 1 2 2 2
  line L62 (-1.182, 4.5084) -> (-1.182, 4.3496)
  line L63 (-1.182, 4.3496) -> (-1.1901, 4.3496)
  spline S15 degree 2 poles (-1.1901, 4.3496) (-1.2282, 4.3934) (-1.3473, 4.4582) (-1.413, 4.4582) knots 0 0 0 1 2 2 2
  spline S16 degree 2 poles (-1.413, 4.4582) (-1.4875, 4.4582) (-1.5791, 4.3715) (-1.5791, 4.301) knots 0 0 0 1 2 2 2
  spline S17 degree 2 poles (-1.5791, 4.301) (-1.5791, 4.2378) (-1.5248, 4.1624) (-1.4737, 4.1454) knots 0 0 0 1 2 2 2
  spline S18 degree 2 poles (-1.4737, 4.1454) (-1.4405, 4.134) (-1.3425, 4.1049) (-1.31, 4.0927) knots 0 0 0 1 2 2 2
  spline S19 degree 2 poles (-1.31, 4.0927) (-1.2274, 4.0611) (-1.1512, 3.9339) (-1.1512, 3.8407) knots 0 0 0 1 2 2 2
  spline S20 degree 2 poles (-1.1512, 3.8407) (-1.1512, 3.7815) (-1.1893, 3.6681) (-1.2233, 3.6284) knots 0 0 0 1 2 2 2
  spline S21 degree 2 poles (-1.2233, 3.6284) (-1.2622, 3.5846) (-1.3595, 3.5376) (-1.4324, 3.5376) knots 0 0 0 1 2 2 2
  spline S22 degree 2 poles (-0.7614, 3.9395) (-0.7614, 3.7321) (-0.8676, 3.4177) (-0.9616, 3.2791) knots 0 0 0 1 2 2 2
  line L64 (-0.9616, 3.2791) -> (-1.0848, 3.2791)
  line L65 (-1.0848, 3.2791) -> (-1.0848, 3.2856)
  spline S23 degree 2 poles (-1.0848, 3.2856) (-1.0434, 3.3318) (-0.96, 3.4671) (-0.9284, 3.5481) knots 0 0 0 1 2 2 2
  spline S24 degree 2 poles (-0.9284, 3.5481) (-0.8951, 3.6348) (-0.8562, 3.8277) (-0.8562, 3.9395) knots 0 0 0 1 2 2 2
  spline S25 degree 2 poles (-0.8562, 3.9395) (-0.8562, 4.0506) (-0.8959, 4.2475) (-0.9284, 4.331) knots 0 0 0 1 2 2 2
  spline S26 degree 2 poles (-0.9284, 4.331) (-0.9616, 4.4144) (-1.0442, 4.5473) (-1.0848, 4.5935) knots 0 0 0 1 2 2 2
  line L66 (-1.0848, 4.5935) -> (-1.0848, 4.6)
  line L67 (-1.0848, 4.6) -> (-0.9616, 4.6)
  spline S27 degree 2 poles (-0.9616, 4.6) (-0.8684, 4.4614) (-0.7614, 4.1486) (-0.7614, 3.9395) knots 0 0 0 1 2 2 2
  point P0 (0, 0)
  dimension "d122" = 0.5
  dimension "d123" = 4.5
  constraints: 2 other
  measures "d122" distance between parallel lines of L4 L0
  measures "d123" distance between parallel lines of L5 L3
extrude "Extrusion15" add sketch "Sketch16" along normal blind 0.1 bodies 6
sketch "Sketch18" plane through (-7.8, -5.1, 1.6) normal (1, 0, 0) x (0, 0, -1)
  arc A0 (0.95, -3.75) -> (2.25, -3.75) centre (1.6, -3.75) ccw projected
sketch "Sketch19" plane through (-0.5, -5.1, 1.6) normal (1, 0, 0) x (0, 0, -1)
  arc A0 (0.95, -3.75) -> (2.25, -3.75) centre (1.6, -3.75) ccw projected
sketch "Sketch20" plane through (8.4, -5.1, 1.6) normal (1, 0, 0) x (0, 0, -1)
  arc A0 (0.95, -3.75) -> (2.25, -3.75) centre (1.6, -3.75) ccw projected
body "Solid2"
body "Solid3"
body "Srf1"
body "Solid4"
body "Solid5"
body "Solid6"
